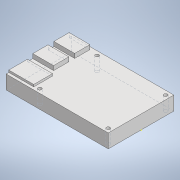
# Autodesk Inventor part: RaspPi_Model
Saved by Autodesk Inventor 2021 (Build 250183000, 183)
## iProperties
Created: 2020-07-08
Part Number: RaspPi_Model
Material: Generic
Document SubType Name: Modeling
Designer: ameli
Density: 1 g/cm^3
Appearance: Default
Author: ameli
Autodesk Inventor part; units mm, degrees
ref_plane "YZ Plane" through (0, 0, 0) normal (1, 0, 0) x (0, 1, 0)
ref_plane "XZ Plane" through (0, 0, 0) normal (0, 1, 0) x (-1, 0, 0)
ref_plane "XY Plane" through (0, 0, 0) normal (0, 0, 1) x (1, 0, 0)
sketch "Sketch1" plane through (0, 0, 0) normal (0, 1, 0) x (-1, 0, 0)
  line L0 (43.575, 28.025) -> (-43.575, 28.025)
  line L1 (-43.575, 28.025) -> (-43.575, -27.975)
  line L2 (-43.575, -27.975) -> (43.575, -27.975)
  line L3 (43.575, -27.975) -> (43.575, 28.025)
  point P0 (0, 0)
  dimension "d0" = 87.15
  dimension "d1" = 56
  dimension "d2" = 27.975
  dimension "d3" = 43.575
  constraints: 8 end point, 2 parallel, 1 horizontal, 1 perpendicular
  measures "d0" distance of L1.end L2.end
  measures "d1" distance of L0.end L1.end
  measures "d2" distance from line of point (0, 0) L2
  measures "d3" distance from line of point (0, 0) L1
extrude "Extrusion1" add sketch "Sketch1" along normal blind 11.8
sketch "Sketch4" plane through (0, 11.8, 0) normal (0, 1, 0) x (1, 0, 0)
  line L0 (-43.575, 25.725) -> (-25.825, 25.725)
  line L1 (-25.825, 25.725) -> (-25.825, 12.725)
  line L2 (-25.825, 12.725) -> (-43.575, 12.725)
  line L3 (-43.575, 12.725) -> (-43.575, 25.725)
  line L4 (-43.575, 7.725) -> (-25.825, 7.725)
  line L5 (-25.825, 7.725) -> (-25.825, -5.275)
  line L6 (-25.825, -5.275) -> (-43.575, -5.275)
  line L7 (-43.575, -5.275) -> (-43.575, 7.725)
  line L8 (43.575, 27.975) -> (-43.575, 27.975) projected
  line L9 (-43.575, 27.975) -> (-43.575, -28.025) projected
  point P0 (0, 0)
  dimension "d12" = 17.75
  dimension "d13" = 13
  dimension "d14" = 5
  dimension "d15" = 13
  dimension "d16" = 17.75
  dimension "d43" = 2.25
  constraints: 16 end point, 4 parallel, 2 horizontal, 2 perpendicular, 1 point on line
  measures "d12" distance of L0.start L0.end
  measures "d13" distance of L0.end L1.end
  measures "d14" distance between parallel lines of L4 L2
  measures "d15" distance of L4.end L5.end
  measures "d16" distance of L4.start L4.end
  measures "d43" distance between parallel lines of L8 L0
extrude "Extrusion2" add sketch "Sketch4" along normal blind 3.7
sketch "Sketch6" plane through (0, 11.8, 0) normal (0, 1, 0) x (1, 0, 0)
  line L0 (-43.575, -9.775) -> (-22.275, -9.775)
  line L1 (-22.275, -9.775) -> (-22.275, -25.775)
  line L2 (-22.275, -25.775) -> (-43.575, -25.775)
  line L3 (-43.575, -25.775) -> (-43.575, -9.775)
  line L4 (-43.575, 25.725) -> (-25.825, 25.725) projected
  line L5 (-43.575, 27.975) -> (-43.575, 25.725) projected
  line L6 (-43.575, -5.275) -> (-25.825, -5.275) projected
  point P0 (0, 0)
  dimension "d19" = 16
  dimension "d20" = 21.3
  dimension "d22" = 0
  dimension "d44" = 4.5
  constraints: 8 end point, 2 parallel, 1 horizontal, 1 perpendicular
  measures "d19" distance of L0.end L1.end
  measures "d20" distance of L1.end L2.end
  measures "d22" distance between parallel lines of L3 L5
  measures "d44" distance between parallel lines of L6 L0
extrude "Extrusion3" add sketch "Sketch6" along normal blind 1.8
sketch "Sketch10" plane through (43.575, 0, 28.025) normal (1, 0, 0) x (0, 0, -1)
  point P0 (28.025, 0)
sketch "Sketch11" plane through (0, 11.8, 0) normal (0, 1, 0) x (1, 0, 0)
  circle A0 centre (-18.425, -24.525) radius 1.5
  circle A1 centre (-18.425, 24.475) radius 1.5
  circle A2 centre (40.075, -24.525) radius 1.5
  circle A3 centre (40.075, 24.475) radius 1.5
  line L0 (-43.575, -5.275) -> (-43.575, -9.775) projected
  line L1 (-43.575, 27.975) -> (-43.575, 25.725) projected
  line L2 (-43.575, -28.025) -> (43.575, -28.025) projected
  line L3 (43.575, -28.025) -> (43.575, 27.975) projected
  line L4 (43.575, 27.975) -> (-43.575, 27.975) projected
  point P0 (0, 0)
  dimension "d45" = 3
  dimension "d46" = 3
  dimension "d47" = 3
  dimension "d48" = 3
  dimension "d50" = 58.5
  dimension "d51" = 58.5
  dimension "d55" = 3.5
  dimension "d56" = 3.5
  dimension "d59" = 3.5
  dimension "d60" = 3.5
  dimension "d61" = 3.5
  dimension "d62" = 3.5
  constraints: 4 centre point
  measures "d45" diameter of A0
  measures "d46" diameter of A1
  measures "d47" diameter of A3
  measures "d48" diameter of A2
  measures "d50" distance of A2.centre A0.centre
  measures "d51" distance of A1.centre A3.centre
  measures "d55" distance from line of L2 A0.centre
  measures "d56" distance from line of L2 A2.centre
  measures "d59" distance from line of L3 A2.centre
  measures "d60" distance from line of L3 A3.centre
  measures "d61" distance from line of L4 A3.centre
  measures "d62" distance from line of L4 A1.centre
extrude "Extrusion7" cut sketch "Sketch11" against normal through all
body "Solid1"
